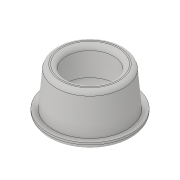
# Autodesk Inventor part: FED ttl plug
Saved by Autodesk Inventor 2017 (Build 210142000, 142)
## iProperties
Part Number: FED ttl plug
Material: Generisch
Document SubType Name: Modeling
Designer: Werkstatt
Density: 1 g/cm^3
Appearance: Vorgabe
Author: Werkstatt
Autodesk Inventor part; units mm, degrees
ref_plane "YZ Plane" through (0, 0, 0) normal (1, 0, 0) x (0, 1, 0)
ref_plane "XZ Plane" through (0, 0, 0) normal (0, 1, 0) x (-1, 0, 0)
ref_plane "XY Plane" through (0, 0, 0) normal (0, 0, 1) x (1, 0, 0)
sketch "Skizze1" plane through (0, 0, 0) normal (0, 1, 0) x (-1, 0, 0)
  line L0 (0, 0) -> (6.5, 0)
  line L1 (6.5, 0) -> (6.5, 1)
  line L2 (6.5, 1) -> (5.7, 1)
  line L3 (5.7, 1) -> (5.1751, 7)
  line L4 (5.1751, 7) -> (0, 7)
  line L5 (0, 7) -> (0, 0)
  line L6 (0, -2.278) -> (0, 8.6565) construction
  dimension "d0" = 6.5
  dimension "d1" = 1
  dimension "d2" = 7
  dimension "d3" = 95
  dimension "d4" = 5.7
  constraints: 14 end point, 3 perpendicular, 1 horizontal, 1 parallel, 1 point on line, 1 vertical
  measures "d0" distance between parallel lines of L6 L1
  measures "d1" distance between parallel lines of L2 L0
  measures "d2" distance between parallel lines of L4 L0
  measures "d3" angle of L4 L3
  measures "d4" distance from line of L5 L2.end
revolve "Umdrehung1" add sketch "Skizze1" angle 360 about axis through (0, 0, -2.278) along (0, 0, 1)
fillet "Rundung1" radius 0.7 1 edges at (6.5, 0, 0)
shell "Wandung1" thickness 1.6 removed faces 1 at (1.38, 0.4128, 7)
fillet "Rundung2" radius 0.7 3 edges at (5.1751, 0, 7) (3.569, 0, 7) (4.0414, 0, 1.6)
